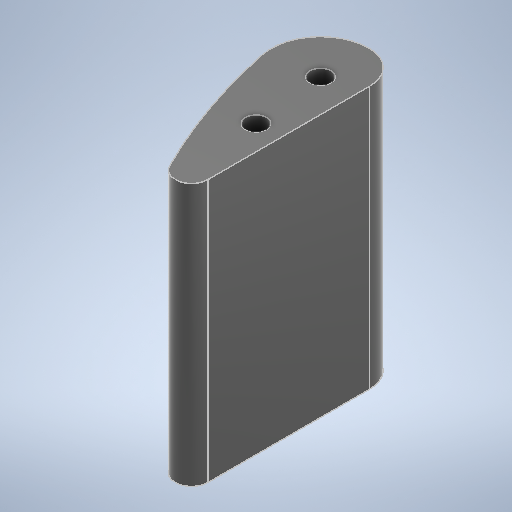
# Autodesk Inventor part: RT_FRM_V2_MC_004_IntermediateB_DynamicsPlate
Saved by Autodesk Inventor 2025.3 (Build 293356000, 356)
## iProperties
Created: 2026-04-28
Part Number: RT_FRM_V2_MC_004_IntermediateB_DynamicsPlate
Material: ABS Plastic
Document SubType Name: Modeling
Designer: louis
Density: 1.06 g/cm^3
Appearance: Smooth - Black
Mass: 556.266 g
Surface Area: 1307.88 cm^2
Volume: 556.266 cm^3
Author: louis
Autodesk Inventor part; units mm, degrees
ref_plane "YZ Plane" through (0, 0, 0) normal (1, 0, 0) x (0, 1, 0)
ref_plane "XZ Plane" through (0, 0, 0) normal (0, 1, 0) x (-1, 0, 0)
ref_plane "XY Plane" through (0, 0, 0) normal (0, 0, 1) x (1, 0, 0)
sketch "Sketch1" plane through (0, 0, 0) normal (0, 1, 0) x (-1, 0, 0)
  line L0 (30, -2.5) -> (140, -2.5)
  line L1 (185, 0) -> (25, 0)
  line L2 (0, 0) -> (25, 0)
  circle A0 centre (0, 0) radius 175
  line L3 (50, 0) -> (103.8137, 0) construction
  line L4 (105, 16.5) -> (105, 0) construction
  line L5 (105, 66.5) -> (105, 16.5) construction
  line L6 (174.1228, -17.5) -> (70, -17.5)
  line L7 (70, -17.5) -> (70, 17.5)
  line L8 (70, 17.5) -> (174.1228, 17.5)
  line L9 (174.1228, 17.5) -> (174.1228, -17.5)
  line L10 (0, 0) -> (0, 175)
  line L11 (-64.9519, 112.5) -> (0, 0)
  circle A1 centre (0, 0) radius 310 construction
  line L12 (-310, -390) -> (-310, -310) construction
  line L13 (-310, -310) -> (-390, -310) construction
  line L14 (-390, -310) -> (-390, -390) construction
  line L15 (-390, -390) -> (-310, -390) construction
  line L16 (-310, -390) -> (-390, -310) construction
  line L17 (-310, -310) -> (-390, -390) construction
  line L18 (-310, 310) -> (-310, 390) construction
  line L19 (-310, 390) -> (-390, 390) construction
  line L20 (-390, 390) -> (-390, 310) construction
  line L21 (-390, 310) -> (-310, 310) construction
  line L22 (-310, 310) -> (-390, 390) construction
  line L23 (-310, 390) -> (-390, 310) construction
  line L24 (390, 310) -> (390, 390) construction
  line L25 (390, 390) -> (310, 390) construction
  line L26 (310, 390) -> (310, 310) construction
  line L27 (310, 310) -> (390, 310) construction
  line L28 (390, 310) -> (310, 390) construction
  line L29 (390, 390) -> (310, 310) construction
  line L30 (390, -390) -> (390, -310) construction
  line L31 (390, -310) -> (310, -310) construction
  line L32 (310, -310) -> (310, -390) construction
  line L33 (310, -390) -> (390, -390) construction
  line L34 (390, -390) -> (310, -310) construction
  line L35 (390, -310) -> (310, -390) construction
  line L36 (310, -310) -> (310, 310) construction
  line L37 (310, 310) -> (-310, 310) construction
  line L38 (-310, 310) -> (-310, -310) construction
  line L39 (-310, -310) -> (310, -310) construction
  line L40 (-64.9519, 112.5) -> (-87.5, 151.5544)
  line L41 (160, 17.5) -> (174.1228, 17.5)
  line L42 (-102.2168, 142.0448) -> (-71.906, 159.5448)
  line L43 (-71.906, -159.5448) -> (-102.2168, -142.0448)
  point P0 (161.4582, -67.5)
  point P1 (70, 0)
  point P2 (-71.906, 159.5448)
  point P3 (-87.0614, 150.7948)
  point P4 (174.1228, 0)
  point P5 (-102.2168, 142.0448)
  point P6 (-71.906, -159.5448)
  point P7 (-102.2168, -142.0448)
  dimension "d0" = 110
  dimension "d2" = 2.5
  dimension "d4" = 105
  dimension "d9" = 350
  dimension "d26" = 35
  dimension "d27" = 35
  dimension "d40" = 50
  dimension "d46" = 120
  dimension "d74" = 80
  dimension "d75" = 80
  dimension "d78" = 80
  dimension "d79" = 80
  dimension "d80" = 80
  dimension "d81" = 80
  dimension "d82" = 80
  dimension "d83" = 80
  dimension "d86" = 620
  dimension "d97" = 360
  constraints: 88 end point, 10 parallel, 10 perpendicular, 6 vertical, 5 point on circle, 3 coincident, 3 horizontal, 3 point on line, 3 tangent, 2 centre point, 2 collinear, 1 midpoint, 10 other
  measures "d0" distance of L0.end L0.start
  measures "d2" distance between parallel lines of L0 L1
  measures "d4" distance of L2.start L4.end
  measures "d9" diameter of A0
  measures "d26" distance between parallel lines of L8 L6
  measures "d27" distance between parallel lines of L4 L7
  measures "d40" distance from line of L6 point (161.458, -67.5)
  measures "d46" angle of L11 L2
  measures "d74" distance of L13.end L14.end
  measures "d75" distance of L14.end L12.start
  measures "d78" distance of L19.end L20.end
  measures "d79" distance of L20.end L18.start
  measures "d80" distance of L25.end L26.end
  measures "d81" distance of L26.end L24.start
  measures "d82" distance of L31.end L32.end
  measures "d83" distance of L32.end L30.start
  measures "d86" distance of L26.end L18.start
extrude "Extrusion1" add sketch "Sketch1" against normal blind 10 contours L8 L7 L1 L2 L10 A0 | L10 L11 L40 L42 A0 | A0 L43
pattern_circular "Circular Pattern2" count 3 over 360 about axis through (0, 0, 0) along (0, -1, 0) of "Extrusion1"
extrude "Extrusion2" cut sketch "Sketch1" against normal blind 10 contours A0 L9 L1 | L1 L9 A0 | L9 L6 L7 L1 | L1 L7 L8 L9
pattern_circular "Circular Pattern1" count 3 over 360 about axis through (0, -10, 0) along (0, 1, 0) of "Extrusion2"
fillet "Fillet1" radius 10 6 edges at (19.8446, -5, 69.3718) (50.1554, -5, -51.8718) (-70, -5, -17.5) (-70, -5, 17.5) (50.1554, -5, 51.8718) (19.8446, -5, -69.3718)
sketch "Sketch2" plane through (0, -10, 0) normal (0, 1, 0) x (1, 0, 0)
  line L0 (20, 310) -> (-20, 310) construction
  line L1 (-20, 310) -> (-20, -310) construction
  line L2 (-20, -310) -> (20, -310) construction
  line L3 (20, -310) -> (20, 310) construction
  line L4 (20, 310) -> (-20, -310) construction
  line L5 (-20, 310) -> (20, -310) construction
  line L6 (60, 20) -> (20, 20) construction
  line L7 (20, 20) -> (20, -20) construction
  line L8 (20, -20) -> (60, -20) construction
  line L9 (60, -20) -> (60, 20) construction
  line L10 (60, 20) -> (20, -20) construction
  line L11 (20, 20) -> (60, -20) construction
  line L12 (-60, 123.6771) -> (-20, 123.6771) construction
  line L13 (-20, 123.6771) -> (-20, 83.6771) construction
  line L14 (-20, 83.6771) -> (-60, 83.6771) construction
  line L15 (-60, 83.6771) -> (-60, 123.6771) construction
  line L16 (-60, 123.6771) -> (-20, 83.6771) construction
  line L17 (-20, 123.6771) -> (-60, 83.6771) construction
  line L18 (-60, -66.8914) -> (-20, -66.8914) construction
  line L19 (-20, -66.8914) -> (-20, -106.8914) construction
  line L20 (-20, -106.8914) -> (-60, -106.8914) construction
  line L21 (-60, -106.8914) -> (-60, -66.8914) construction
  line L22 (-60, -66.8914) -> (-20, -106.8914) construction
  line L23 (-20, -66.8914) -> (-60, -106.8914) construction
  point P0 (0, 0)
  point P1 (40, 0)
  point P2 (-40, 103.6771)
  point P3 (-40, -86.8914)
  dimension "d87" = 40
  dimension "d88" = 620
  dimension "d89" = 40
  dimension "d90" = 40
  dimension "d91" = 40
  dimension "d92" = 40
  dimension "d93" = 40
  dimension "d94" = 40
  constraints: 48 end point, 8 midpoint, 8 parallel, 4 horizontal, 4 perpendicular, 3 collinear
  measures "d87" distance of L2.end L1.end
  measures "d88" distance of L1.end L0.end
  measures "d89" distance of L8.end L7.end
  measures "d90" distance of L7.end L6.end
  measures "d91" distance of L13.end L14.end
  measures "d92" distance of L19.end L20.end
  measures "d93" distance of L18.end L19.end
  measures "d94" distance of L14.end L12.start
hole "Hole2" [suppressed]
sketch "Sketch3" plane through (0, -10, 0) normal (0, -1, 0) x (1, 0, 0)
  point P0 (0, 0)
  point P1 (0, 0)
  constraints: 1 coincident
hole "Hole3" at (0, -10, 0) direction (0, 1, 0) diameter 6.6 end through all counterbore diameter 11 counterbore depth 6 clearance for "Socket Head Cap Screw" size "M6" standard "Ansi Metric M Profile"
fillet "Fillet2" radius 15 6 edges at (71.906, -5, -159.5448) (102.2168, -5, -142.0448) (102.2168, -5, 142.0448) (71.906, -5, 159.5448) (-174.1228, -5, -17.5) (-174.1228, -5, 17.5)
sketch "Sketch4" plane through (0, -10, 0) normal (0, 1, 0) x (1, 0, 0)
  line L0 (-20, -310) -> (20, -310) construction
  line L1 (20, -310) -> (20, 310) construction
  line L2 (20, 310) -> (-20, 310) construction
  line L3 (-20, 310) -> (-20, -310) construction
  circle A0 centre (0, 0) radius 3.3 construction
  line L4 (-20, -310) -> (20, 310) construction
  line L5 (20, -310) -> (-20, 310) construction
  line L6 (-55, 117.5) -> (-20, 117.5) construction
  line L7 (-20, 117.5) -> (-20, 82.5) construction
  line L8 (-20, 82.5) -> (-55, 82.5) construction
  line L9 (-55, 82.5) -> (-55, 117.5) construction
  line L10 (-55, 117.5) -> (-20, 82.5) construction
  line L11 (-20, 117.5) -> (-55, 82.5) construction
  line L12 (20, 17.5) -> (55, 17.5) construction
  line L13 (55, 17.5) -> (55, -17.5) construction
  line L14 (55, -17.5) -> (20, -17.5) construction
  line L15 (20, -17.5) -> (20, 17.5) construction
  line L16 (20, 17.5) -> (55, -17.5) construction
  line L17 (55, 17.5) -> (20, -17.5) construction
  line L18 (-55, -82.5) -> (-20, -82.5) construction
  line L19 (-20, -82.5) -> (-20, -117.5) construction
  line L20 (-20, -117.5) -> (-55, -117.5) construction
  line L21 (-55, -117.5) -> (-55, -82.5) construction
  line L22 (-55, -82.5) -> (-20, -117.5) construction
  line L23 (-20, -82.5) -> (-55, -117.5) construction
  line L24 (0, 0) -> (37.5, 0) construction
  line L25 (-37.5, 100) -> (-37.5, -100) construction
  line L26 (-37.5, 0) -> (0, 0) construction
  point P0 (37.5, 0)
  dimension "d113" = 40
  dimension "d114" = 620
  dimension "d115" = 35
  dimension "d116" = 35
  dimension "d117" = 35
  dimension "d118" = 35
  dimension "d119" = 35
  dimension "d120" = 35
  dimension "d121" = 200
  constraints: 54 end point, 9 midpoint, 8 parallel, 5 horizontal, 5 perpendicular, 3 coincident, 3 collinear
  measures "d113" distance of L2.end L1.end
  measures "d114" distance of L1.end L0.end
  measures "d115" distance of L7.end L8.end
  measures "d116" distance of L6.end L7.end
  measures "d117" distance of L13.end L14.end
  measures "d118" distance of L12.end L13.end
  measures "d119" distance of L19.end L20.end
  measures "d120" distance of L18.end L19.end
  measures "d121" distance of L25.start L25.end
hole "Hole4" at (-37.5, -10, -100) at (-37.5, -10, 100) at (37.5, -10, 0) direction (0, 1, 0) diameter 6.6 end through all counterbore diameter 11 counterbore depth 6 clearance for "Socket Head Cap Screw" size "M6" standard "Ansi Metric M Profile"
sketch "Sketch5" plane through (0, 0, 0) normal (0, -1, 0) x (1, 0, 0)
  circle A0 centre (0, 0) radius 175
  arc A1 (63.1768, 144.4254) -> (54.8914, 166.1684) centre (50.1864, 151.9254) ccw projected
  circle A2 centre (50.1864, 151.9254) radius 15
  arc A3 (54.8914, 166.1684) -> (-171.3517, 35.5469) centre (0, 0) ccw projected
  line L0 (24.8446, 78.032) -> (63.1768, 144.4254) projected
  circle A4 centre (0, 0) radius 3.3 projected
  circle A5 centre (0, 0) radius 60
  line L1 (63.1768, 144.4254) -> (13.5402, 58.4522)
  line L2 (-70, -7.5) -> (-70, 7.5) projected
  line L3 (-70, 0) -> (-70, 160.3901)
  circle A6 centre (-55, 50.9902) radius 15
  circle A7 centre (5.6504, 74.7868) radius 15
  circle A8 centre (-55, 150.2498) radius 15
  line L4 (50.1864, 151.9254) -> (-55, 150.2498) construction
  line L5 (-55, 150.2498) -> (-55, 50.9902) construction
  line L6 (-55, 50.9902) -> (5.6504, 74.7868) construction
  line L7 (5.6504, 74.7868) -> (50.1864, 151.9254) construction
  line L8 (-80, 17.5) -> (-156.6645, 17.5) projected
  arc A9 (-171.3517, 35.5469) -> (-156.6645, 17.5) centre (-156.6645, 32.5) ccw projected
  arc A10 (-156.6645, 17.5) -> (-146.6645, 27.5) centre (-156.6645, 27.5) ccw
  line L9 (-146.6645, 27.5) -> (-146.6645, 95.4701)
  circle A11 centre (-151.6645, 76.7978) radius 5
  arc A12 (54.8914, 166.1684) -> (-171.3517, 35.5469) centre (0, 0) ccw projected
  line L10 (-156.6645, 32.5) -> (-151.6645, 76.7978) construction
  circle A13 centre (0, 0) radius 160 construction
  line L11 (-2.4068, 151.0876) -> (-2.5485, 159.9797) construction
  point P0 (-24.6748, 62.8885)
  point P1 (27.9184, 113.3561)
  point P2 (-55, 100.62)
  point P3 (-154.1645, 54.6489)
  point P4 (-70, 150.2498)
  point P5 (-70, 50.9902)
  point P6 (-44, 40.7922)
  point P7 (4.5204, 59.8295)
  point P8 (18.6408, 67.2868)
  point P9 (-60.1562, 164.3357)
  point P10 (-146.6645, 76.7978)
  point P11 (-156.1252, 79.0565)
  dimension "d130" = 120
  dimension "d129" = 350
  dimension "d131" = 30
  dimension "d132" = 30
  dimension "d133" = 30
  dimension "d148" = 10
  dimension "d149" = 10
  constraints: 18 end point, 8 coincident, 8 tangent, 7 centre point, 6 midpoint, 6 point on circle, 2 vertical, 1 perpendicular, 1 point on line, 10 other
  measures "d129" diameter of A0
  measures "d131" diameter of A6
  measures "d132" diameter of A7
  measures "d133" diameter of A8
  measures "d148" radius of A10
  measures "d149" diameter of A11
hole "Hole5" at (27.9184, 0, 113.3561) at (50.1864, 0, 151.9254) at (-55, 0, 150.2498) at (-156.6645, 0, 32.5) at (-154.1645, 0, 54.6489) at (-24.6748, 0, 62.8885) direction (0, -1, 0) diameter 5.5 end through all countersink diameter 10.4 countersink angle 90 clearance for "Flat Head Machine Screw" size "M5" standard "Ansi Metric M Profile"
pattern_circular "Circular Pattern4" count 3 over 360 about axis through (0, 484.456, 0) along (0, -1, 0) of "Hole5"
extrude "Extrusion4" add sketch "Sketch5" against normal blind 80 separate body contours A0 A11 L9 A10 A9 | A11
hole "Hole6" at (-154.1645, 0, 54.6489) at (-156.6645, 0, 32.5) direction (0, 1, 0) diameter 6.4 end through all
body "Solid1"
body "Solid2"
